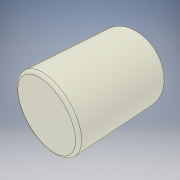
# Autodesk Inventor part: 2P1-2TB-B201A-Z_button_circle
Saved by Autodesk Inventor 2018 (Build 220112000, 112)
## iProperties
Created: 2021-02-02
Part Number: 2P1-2TB-B201A-Z_button_circle
Material: Všeobecné
Document SubType Name: Modeling
Designer: Jozko Mrkvicka
Density: 1 g/cm^3
Appearance: Výchozí
Author: Jozko Mrkvicka
Autodesk Inventor part; units mm, degrees
ref_plane "YZ Plane" through (0, 0, 0) normal (1, 0, 0) x (0, 1, 0)
ref_plane "XZ Plane" through (0, 0, 0) normal (0, 1, 0) x (-1, 0, 0)
ref_plane "XY Plane" through (0, 0, 0) normal (0, 0, 1) x (1, 0, 0)
sketch "Náčrt1" plane through (0, 0, 0) normal (0, 1, 0) x (-1, 0, 0)
  circle A0 centre (0, 0) radius 3.4925
  dimension "d0" = 6.985
  constraints: 1 centre point, 1 coincident
  measures "d0" diameter of A0
extrude "Vysunutí1" add sketch "Náčrt1" along normal blind 8.255
chamfer "Zkosení1" distance 0.3175 distance2 8.255 1 edges at (3.4925, 8.255, 0) measured on face at (-1.152, 8.255, -0.772)
sketch "Náčrt2" plane through (0, 0, 0) normal (0, -1, 0) x (1, 0, 0)
  circle A0 centre (0, 0) radius 3.4925 projected
  line L0 (1.905, -1.905) -> (-1.905, 1.905) construction
  line L1 (-1.905, -1.905) -> (1.905, 1.905) construction
  line L2 (-0.635, 1.905) -> (-0.635, 1.27)
  line L3 (-0.635, 1.27) -> (0.635, 1.27)
  line L4 (0.635, 1.27) -> (0.635, 1.905)
  line L5 (-0.635, -1.905) -> (-0.635, -1.2721)
  line L6 (-0.635, -1.2721) -> (0.635, -1.2721)
  line L7 (0.635, -1.2721) -> (0.635, -1.905)
  line L8 (-1.905, -0.6371) -> (-1.2679, -0.6371)
  line L9 (-1.2679, -0.6371) -> (-1.2679, 0.6371)
  line L10 (-1.2679, 0.6371) -> (-1.905, 0.6371)
  line L11 (1.905, -0.6371) -> (1.2679, -0.6371)
  line L12 (1.2679, -0.6371) -> (1.2679, 0.6371)
  line L13 (1.2679, 0.6371) -> (1.905, 0.6371)
  line L14 (-1.905, -1.905) -> (-1.905, -0.6371)
  line L15 (-1.905, 0.6371) -> (-1.905, 1.905)
  line L16 (-1.905, 1.905) -> (-0.635, 1.905)
  line L17 (0.635, 1.905) -> (1.905, 1.905)
  line L18 (1.905, -1.905) -> (0.635, -1.905)
  line L19 (-0.635, -1.905) -> (-1.905, -1.905)
  line L20 (1.905, 1.905) -> (1.905, 0.6371)
  line L21 (1.905, -0.6371) -> (1.905, -1.905)
  dimension "d6" = 3.81
  dimension "d7" = 3.81
  constraints: 44 end point, 12 parallel, 6 perpendicular, 4 horizontal, 2 midpoint, 2 point on line
  measures "d6" distance of L0.end L1.end
  measures "d7" distance of L1.start L0.end
extrude "Vysunutí2" cut sketch "Náčrt2" against normal blind 7.62 contours L2 L3 L4 L17 L20 L13 L12 L11 L21 L18 L7 L6 L5 L19 L14 L8 L9 L10 L15 L16
fillet "Zaoblení1" radius 0.254 1 edges at (3.1755, 8.255, 0)
